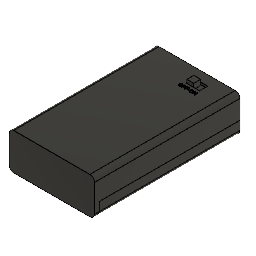
727 3xAAA JST Battery Holder (Autodesk Fusion 360 design; units mm, degrees)
Autodesk Fusion 360 part; units mm, degrees
sketch "base" plane through (0, 0, 0) normal (0, 0, 1) x (1, 0, 0)
  line L0 (0, 0) -> (37, 0)
  line L1 (37, 0) -> (37, 63)
  line L2 (37, 63) -> (0, 63)
  line L3 (0, 63) -> (0, 0)
  dimension "d1" = 37
  dimension "d2" = 63
extrude "Extrude1" add sketch "base" along normal blind 16 makes body 1
fillet "Fillet1" radius 2 4 edges at (37, 31.5, 16) (37, 31.5, 0) (0, 31.5, 16) (0, 31.5, 0) on bodies 1
ref_plane "WorkPlane1" through (18.5, 31.5, 16) normal (0, 0, 1) x (1, 0, 0)
sketch "switch hole" plane through (18.5, 31.5, 16) normal (0, 0, 1) x (1, 0, 0)
  line L0 (2.9, 27.1) -> (8.9, 27.1)
  line L1 (8.9, 27.1) -> (8.9, 23.6)
  line L2 (8.9, 23.6) -> (2.9, 23.6)
  line L3 (2.9, 23.6) -> (2.9, 27.1)
  line L4 (18.5, -31.5) -> (18.5, 31.5)
  line L5 (18.5, 31.5) -> (18.5, -31.5)
  line L6 (16.5, 31.5) -> (-16.5, 31.5)
  dimension "d7" = 6
  dimension "d8" = 3.5
  dimension "d9" = 4.4
  dimension "d10" = 9.6
  measures "d9" distance of L0 L6
  measures "d10" distance of L1
extrude "Extrude2" cut sketch "switch hole" against normal blind 1 bodies 1
sketch "switch actuator" plane through (0, 0, 15) normal (0, 0, 1) x (-1, 0, 0)
  line L0 (-21.4, -55.1) -> (-27.4, -55.1)
  line L1 (-27.4, -55.1) -> (-27.4, -58.6)
  line L2 (-27.4, -58.6) -> (-21.4, -58.6)
  line L3 (-21.4, -58.6) -> (-21.4, -55.1)
  line L4 (-21.65, -55.35) -> (-24.65, -55.35)
  line L5 (-24.65, -55.35) -> (-24.65, -58.35)
  line L6 (-24.65, -58.35) -> (-21.65, -58.35)
  line L7 (-21.65, -58.35) -> (-21.65, -55.35)
  line L8 (-21.4, -55.1) -> (-21.4, -58.6)
  line L9 (-27.4, -55.1) -> (-21.4, -55.1)
  line L10 (-21.65, -56.85) -> (-21.4, -56.85)
  dimension "d13" = 3
  dimension "d14" = 3
  dimension "d17" = 0.25
extrude "Extrude3" add sketch "switch actuator" along normal blind 2.3 contours L4 L5 L6 L7 bodies 1
sketch "wire hole" plane through (0, 63, 0) normal (0, 1, 0) x (-1, 0, 0)
  arc A0 (-2, 0) -> (0, 2) centre (-2, 2) ccw
  line L0 (0, 2) -> (0, 14)
  arc A1 (0, 14) -> (-2, 16) centre (-2, 14) ccw
  line L1 (-2, 16) -> (-35, 16)
  arc A2 (-35, 16) -> (-37, 14) centre (-35, 14) ccw
  line L2 (-37, 14) -> (-37, 2)
  arc A3 (-37, 2) -> (-35, 0) centre (-35, 2) ccw
  line L3 (-35, 0) -> (-2, 0)
  circle A4 centre (-4.4, 9.6) radius 2
  dimension "d20" = 4
  dimension "d21" = 6.4
  dimension "d22" = 4.4
  measures "d20" diameter of A4
  measures "d21" distance of L1
  measures "d22" distance of L0
extrude "Extrude4" cut sketch "wire hole" against normal blind 2 contours A4 bodies 1
sketch "splitter" plane through (0, 0, 0) normal (1, 0, 0) x (0, 1, 0)
  line L0 (63, 0) -> (0, 0)
  line L1 (2, -5.6898) -> (2, 5.8)
  line L2 (63, 2) -> (63, 14)
  line L3 (2, 5.8) -> (65, 5.8)
  line L4 (2, -5.6898) -> (65, -5.6898)
  line L5 (65, -5.6898) -> (65, 5.8)
  dimension "d25" = 2
  dimension "d26" = 5.8
  measures "d25" distance of L1 L0.end
  measures "d26" distance of L3 L0.end
split "Split1" by curves path "splitter" along L3 L1 L4 L5 bodies 1 makes body 2 at (19.4667, 18.3667, 16)
sketch "mhole" plane through (0, 0, 0) normal (0, 0, 1) x (1, 0, 0)
  circle A0 centre (10.5, 57.6) radius 1.9
  circle A1 centre (10.5, 57.6) radius 1
  line L0 (35, 63) -> (2, 63)
  line L1 (0, 2) -> (0, 63)
  dimension "d27" = 3.8
  dimension "d28" = 2
  dimension "d34" = 5.4
  dimension "d35" = 10.5
  measures "d27" diameter of A0
  measures "d28" diameter of A1
  measures "d34" distance of L0
  measures "d35" distance of L1
extrude "Extrude5" cut sketch "mhole" along normal blind 1 contours A0 | A1 bodies 1
extrude "Extrude6" cut sketch "mhole" along normal blind 2 from surface at 1 contours A1 bodies 1
sketch "wires" plane through (0, 61, 0) normal (0, 1, 0) x (-1, 0, 0)
  circle A0 centre (-4.4, 9.6) radius 2
  circle A1 centre (-3.8, 9.6009) radius 0.6
  circle A2 centre (-5, 9.6) radius 0.6
  dimension "d36" = 1.2
  dimension "d37" = 1.2
  dimension "d38" = 1.2
  measures "d36" diameter of A1
  measures "d37" diameter of A2
extrude "Extrude7" add sketch "wires" along normal blind 5 separate body contours A1 | A2 makes body 3 at (5.597, 64.3333, 9.5403)
sketch "text" plane through (0, 0, 16) normal (0, 0, 1) x (-1, 0, 0)
  line L0 (-27.4, -58.6) -> (-27.4, -55.1)
  line L1 (-27.4, -55.1) -> (-21.4, -55.1)
  line L2 (-21.4, -55.1) -> (-21.4, -58.6)
  line L3 (-21.4, -58.6) -> (-27.4, -58.6)
  line L4 (-2, -63) -> (-2, 0)
  line L5 (-2, 0) -> (-35, 0)
  line L6 (-35, 0) -> (-35, -63)
  line L7 (-35, -63) -> (-2, -63)
  line L8 (-20.5294, -52.3242) -> (-27.9337, -52.3242) construction
  line L9 (-27.9337, -52.3242) -> (-27.9337, -54.3242) construction
  line L10 (-27.9337, -54.3242) -> (-20.5294, -54.3242) construction
  line L11 (-20.5294, -54.3242) -> (-20.5294, -52.3242) construction
  text T0 "OFF-ON" font "Arial" height 2 align ink ink in box 0 x 0 at (-20.5394, -52.3442) x (-1, 0) y (0, -1) spacing 1 height is em
extrude "Extrude8" add sketch "text" along normal blind 0.2 text T0 bodies 2
